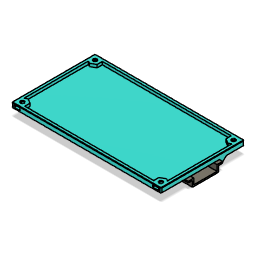
RelayBoardMount (Autodesk Fusion 360 design; units mm, degrees)
Autodesk Fusion 360 part; units mm, degrees
sketch "Skizze1" plane through (0, 0, 0) normal (1, 0, 0) x (0, 0, -1) in component "Rail"
  line L0 (-17.75, 0) -> (17.75, 0)
  line L1 (-13.5, -7.5) -> (13.5, -7.5)
  line L2 (0, -7.5) -> (0, 0) construction
  line L3 (-17.75, 0) -> (-17.75, -1.5)
  line L4 (17.75, 0) -> (17.75, -1.5)
  line L5 (13.5, -7.5) -> (13.5, -1.5)
  line L6 (13.5, -1.5) -> (17.75, -1.5)
  line L7 (-17.75, -1.5) -> (-13.5, -1.5)
  line L8 (-13.5, -1.5) -> (-13.5, -7.5)
  line L9 (-12, 0) -> (-12, -6)
  line L10 (-12, -6) -> (12, -6)
  line L11 (12, -6) -> (12, 0)
  dimension "d1" = 35.5
  dimension "d2" = 27
  dimension "d3" = 1.5
  dimension "d5" = 7.5
  dimension "d6" = 1.5
  dimension "d7" = 1.5
  dimension "d8" = 1.5
  constraint horizontal L0
  constraint midpoint L2.end L0
  constraint horizontal L1
  constraint midpoint L1 L2.start
  constraint coincident L2.end origin
  constraint vertical L2
  constraint perpendicular L0 L3
  constraint perpendicular L0 L4
  constraint perpendicular L1 L5
  constraint perpendicular L4 L6
  constraint perpendicular L5 L7
  constraint perpendicular L7 L8
  constraint equal L3 L4
  constraint coincident L0 L9.start
  constraint perpendicular L0 L9
  constraint perpendicular L5 L10
  constraint coincident L0 L11.end
  constraint perpendicular L0 L11
  measures "d1" distance of L0.start L0.end
  measures "d2" distance of L1.start L1.end
  measures "d3" distance of L0.end L4.end
  measures "d5" distance of L0 L1
  measures "d6" distance of L1 L10
  measures "d7" distance of L8 L9
  measures "d8" distance of L5 L11
extrude "Extrusion1" add sketch "Skizze1" along normal mid plane 160 contours L0 L1 L3 L4 L5 L6 L7 L8 L9 L10 L11 makes body 1 in component "Rail"
sketch "Skizze2" plane through (0, 0, 0) normal (0, 1, 0) x (1, 0, 0) in component "RelayBottom"
  line L0 (-74, 40) -> (74, 40)
  line L1 (74, 40) -> (74, -40)
  line L2 (74, -40) -> (-74, -40)
  line L3 (-74, -40) -> (-74, 40)
  line L4 (-74, 40) -> (74, -40) construction
  line L5 (74, 40) -> (-74, -40) construction
  line L6 (-77, 43) -> (77, 43)
  line L7 (77, 43) -> (77, -43)
  line L8 (77, -43) -> (-77, -43)
  line L9 (-77, -43) -> (-77, 43)
  circle A0 centre (-71.5, 37.5) radius 2
  line L10 (71.5, -37.5) -> (-71.5, -37.5) construction
  line L11 (-71.5, -37.5) -> (-71.5, 37.5) construction
  line L12 (-71.5, 37.5) -> (71.5, 37.5) construction
  line L13 (71.5, 37.5) -> (71.5, -37.5) construction
  line L14 (71.5, -37.5) -> (-71.5, 37.5) construction
  line L15 (-71.5, -37.5) -> (71.5, 37.5) construction
  circle A1 centre (71.5, 37.5) radius 2
  circle A2 centre (71.5, -37.5) radius 2
  circle A3 centre (-71.5, -37.5) radius 2
  line L16 (-68.5, 39.2321) -> (-71.5, 40.9641)
  line L17 (-71.5, 40.9641) -> (-74.5, 39.2321)
  line L18 (-74.5, 39.2321) -> (-74.5, 35.7679)
  line L19 (-74.5, 35.7679) -> (-71.5, 34.0359)
  line L20 (-71.5, 34.0359) -> (-68.5, 35.7679)
  line L21 (-68.5, 35.7679) -> (-68.5, 39.2321)
  line L22 (-68.5, 39.2321) -> (-68.5, 43)
  line L23 (-74.5, 39.2321) -> (-74.5, 43)
  line L24 (74.5, 35.7679) -> (74.5, 39.2321)
  line L25 (74.5, 39.2321) -> (71.5, 40.9641)
  line L26 (71.5, 40.9641) -> (68.5, 39.2321)
  line L27 (68.5, 39.2321) -> (68.5, 35.7679)
  line L28 (68.5, 35.7679) -> (71.5, 34.0359)
  line L29 (71.5, 34.0359) -> (74.5, 35.7679)
  line L30 (74.5, -35.7679) -> (71.5, -34.0359)
  line L31 (71.5, -34.0359) -> (68.5, -35.7679)
  line L32 (68.5, -35.7679) -> (68.5, -39.2321)
  line L33 (68.5, -39.2321) -> (71.5, -40.9641)
  line L34 (71.5, -40.9641) -> (74.5, -39.2321)
  line L35 (74.5, -39.2321) -> (74.5, -35.7679)
  line L36 (-68.5, -35.7679) -> (-71.5, -34.0359)
  line L37 (-71.5, -34.0359) -> (-74.5, -35.7679)
  line L38 (-74.5, -35.7679) -> (-74.5, -39.2321)
  line L39 (-74.5, -39.2321) -> (-71.5, -40.9641)
  line L40 (-71.5, -40.9641) -> (-68.5, -39.2321)
  line L41 (-68.5, -39.2321) -> (-68.5, -35.7679)
  line L42 (-74.5, -39.2321) -> (-74.5, -43)
  line L43 (-68.5, -39.2321) -> (-68.5, -43)
  line L44 (68.5, -39.2321) -> (68.5, -43)
  line L45 (74.5, -39.2321) -> (74.5, -43)
  line L46 (68.5, 39.2321) -> (68.5, 43)
  line L47 (74.5, 39.2321) -> (74.5, 43)
  line L48 (66.5, -39.2321) -> (66.5, -43)
  line L49 (66.5, -34.6132) -> (66.5, -39.2321)
  line L50 (71.5, -31.7265) -> (66.5, -34.6132)
  line L51 (76.5, -34.6132) -> (71.5, -31.7265)
  line L52 (76.5, -39.2321) -> (76.5, -34.6132)
  line L53 (76.5, -39.2321) -> (76.5, -43)
  line L54 (76.5, 39.2321) -> (76.5, 43)
  line L55 (76.5, 34.6132) -> (76.5, 39.2321)
  line L56 (71.5, 31.7265) -> (76.5, 34.6132)
  line L57 (66.5, 34.6132) -> (71.5, 31.7265)
  line L58 (66.5, 39.2321) -> (66.5, 34.6132)
  line L59 (66.5, 39.2321) -> (66.5, 43)
  line L60 (-66.5, 39.2321) -> (-66.5, 43)
  line L61 (-66.5, 34.6132) -> (-66.5, 39.2321)
  line L62 (-71.5, 31.7265) -> (-66.5, 34.6132)
  line L63 (-76.5, 34.6132) -> (-71.5, 31.7265)
  line L64 (-76.5, 39.2321) -> (-76.5, 34.6132)
  line L65 (-76.5, 39.2321) -> (-76.5, 43)
  line L66 (-76.5, -39.2321) -> (-76.5, -43)
  line L67 (-76.5, -34.6132) -> (-76.5, -39.2321)
  line L68 (-71.5, -31.7265) -> (-76.5, -34.6132)
  line L69 (-66.5, -34.6132) -> (-71.5, -31.7265)
  line L70 (-66.5, -39.2321) -> (-66.5, -34.6132)
  line L71 (-66.5, -39.2321) -> (-66.5, -43)
  point P0 (-71.5, 37.5)
  point P1 (71.5, 37.5)
  point P2 (71.5, -37.5)
  point P3 (-71.5, -37.5)
  dimension "d21" = 148
  dimension "d22" = 80
  dimension "d23" = -3
  dimension "d26" = 4
  dimension "d28" = 2.5
  dimension "d29" = 2.5
  dimension "d31" = 6
  dimension "d35" = 2
  dimension "d36" = 2
  dimension "d37" = -2
  dimension "d38" = 2
  constraint horizontal L0
  constraint perpendicular L0 L1
  constraint parallel L0 L2
  constraint parallel L1 L3
  constraint coincident L4 origin
  constraint coincident L5 origin
  constraint horizontal L10
  constraint perpendicular L10 L11
  constraint parallel L10 L12
  constraint parallel L11 L13
  constraint coincident L14 origin
  constraint coincident L15 origin
  constraint coincident P0 A0.centre
  constraint coincident P1 L12.end
  constraint coincident P2 L10.start
  constraint coincident P3 L10.end
  constraint equal A0 A3
  constraint equal A0 A2
  constraint equal A0 A1
  constraint coincident L6 L22.end
  constraint perpendicular L6 L22
  constraint coincident L6 L23.end
  constraint perpendicular L6 L23
  constraint collinear L21 L22
  constraint equal L21 L26
  constraint equal L21 L32
  constraint equal L21 L41
  constraint coincident L8 L42.end
  constraint parallel L38 L42
  constraint perpendicular L8 L42
  constraint coincident L8 L43.end
  constraint perpendicular L8 L43
  constraint coincident L8 L44.end
  constraint perpendicular L8 L44
  constraint collinear L32 L44
  constraint coincident L8 L45.end
  constraint perpendicular L8 L45
  constraint coincident L6 L46.end
  constraint perpendicular L6 L46
  constraint collinear L27 L46
  constraint coincident L6 L47.end
  constraint perpendicular L6 L47
  measures "d21" distance of L1.end L2.end
  measures "d22" distance of L0.end L1.end
  measures "d26" diameter of A0
  measures "d28" distance of L1 L13
  measures "d29" distance of L2 L10
  measures "d31" distance of L18 L21
extrude "Extrusion2" add sketch "Skizze2" along normal blind 2 separate body contours L0 L3 L6 L16 L17 L22 L23 | L0 L3 L17 | L0 L16 L17 | L0 L3 L16 L17 L19 L20 L21 | L3 L17 L18 L19 | L0 L16 L22 | L0 L3 L19 L20 L21 L22 L60 L61 L62 L63 | L3 L6 L18 L19 L23 L63 L64 L65 | L0 L6 L22 L60 | L0 L1 L2 L3 L48 L49 L50 L51 L56 L57 L58 L59 L60 L61 L62 L63 L68 L69 L70 L71 | L3 L6 L8 L9 L63 L64 L65 L66 L67 L68 | L0 L6 L59 L60 | L2 L3 L36 L37 L41 L43 L68 L69 L70 L71 | L3 L8 L37 L38 L42 L66 L67 L68 | L0 L6 L46 L59 | L0 L1 L27 L28 L29 L46 L56 L57 L58 L59 | L2 L3 L36 L37 L39 L40 L41 | L3 L37 L38 L39 | L0 L1 L6 L25 L26 L46 L47 | L0 L26 L46 | L2 L3 L39 | L2 L3 L8 L39 L40 L42 L43 | L0 L25 L26 | L0 L1 L25 L26 L27 L28 L29 | L2 L39 L40 | L0 L1 L25 | L1 L6 L24 L29 L47 L54 L55 L56 | L2 L40 L43 | L2 L8 L43 L71 | L2 L8 L48 L71 | L1 L24 L25 L29 | L1 L6 L7 L8 L51 L52 L53 L54 L55 L56 | L1 L2 L30 L31 L32 L44 L48 L49 L50 L51 | L2 L8 L44 L48 | L1 L8 L30 L35 L45 L51 L52 L53 | L2 L33 L44 | L1 L2 L8 L33 L34 L44 L45 | L1 L30 L34 L35 | L1 L2 L30 L31 L32 L33 L34 | L2 L33 L34 | L1 L2 L34 | A0 | A1 | A2 | A3 makes body 2 in component "RelayBottom"
extrude "Extrusion4" add sketch "Skizze2" along normal blind 3 from surface at 2 contours L0 L3 L6 L16 L17 L22 L23 | L0 L3 L17 | L0 L16 L17 | L0 L3 L16 L17 L19 L20 L21 | L3 L17 L18 L19 | L0 L16 L22 | L0 L3 L19 L20 L21 L22 L60 L61 L62 L63 | L3 L6 L18 L19 L23 L63 L64 L65 | L0 L6 L22 L60 | L3 L6 L8 L9 L63 L64 L65 L66 L67 L68 | L0 L6 L59 L60 | L2 L3 L36 L37 L41 L43 L68 L69 L70 L71 | L3 L8 L37 L38 L42 L66 L67 L68 | L0 L6 L46 L59 | L0 L1 L27 L28 L29 L46 L56 L57 L58 L59 | L2 L3 L36 L37 L39 L40 L41 | L3 L37 L38 L39 | L0 L1 L6 L25 L26 L46 L47 | L0 L26 L46 | L2 L3 L39 | L2 L3 L8 L39 L40 L42 L43 | L0 L25 L26 | L0 L1 L25 L26 L27 L28 L29 | L2 L39 L40 | L0 L1 L25 | L1 L6 L24 L29 L47 L54 L55 L56 | L2 L40 L43 | L2 L8 L43 L71 | L2 L8 L48 L71 | L1 L24 L25 L29 | L1 L6 L7 L8 L51 L52 L53 L54 L55 L56 | L1 L2 L30 L31 L32 L44 L48 L49 L50 L51 | L2 L8 L44 L48 | L1 L8 L30 L35 L45 L51 L52 L53 | L2 L33 L44 | L1 L2 L8 L33 L34 L44 L45 | L1 L30 L34 L35 | L1 L2 L30 L31 L32 L33 L34 | L2 L33 L34 | L1 L2 L34 bodies 2 in component "RelayBottom"
extrude "Extrusion3" cut sketch "Skizze2" along normal blind 2.5 from surface at 1.5 contours L0 L3 L6 L16 L17 L22 L23 | L0 L3 L17 | L0 L16 L17 | L0 L3 L16 L17 L19 L20 L21 | L3 L17 L18 L19 | L0 L16 L22 | L2 L3 L36 L37 L39 L40 L41 | L3 L37 L38 L39 | L0 L1 L6 L25 L26 L46 L47 | L0 L26 L46 | L2 L3 L39 | L2 L3 L8 L39 L40 L42 L43 | L0 L25 L26 | L0 L1 L25 L26 L27 L28 L29 | L2 L39 L40 | L0 L1 L25 | L2 L40 L43 | L1 L24 L25 L29 | L2 L33 L44 | L1 L2 L8 L33 L34 L44 L45 | L1 L30 L34 L35 | L1 L2 L30 L31 L32 L33 L34 | L2 L33 L34 | L1 L2 L34 | A0 | A1 | A2 | A3 bodies 2 in component "RelayBottom"
fillet "Abrundung2" radius 1 4 edges at (-77, 2.5, 43) (77, 2.5, 43) (77, 2.5, -43) (-77, 2.5, -43) on bodies 2 in component "RelayBottom"
sketch "Skizze3" plane through (0, 0, 0) normal (1, 0, 0) x (0, 0, -1) in component "RelayBottom"
  line L0 (-17.75, -1.5) -> (-17.75, 0)
  line L1 (-17.75, 0) -> (-12, 0)
  line L2 (-12, 0) -> (-12, -6)
  line L3 (-12, -6) -> (12, -6)
  line L4 (12, -6) -> (12, 0)
  line L5 (12, 0) -> (17.75, 0)
  line L6 (17.75, 0) -> (17.75, -1.5)
  line L7 (17.75, -1.5) -> (13.5, -1.5)
  line L8 (13.5, -1.5) -> (13.5, -7.5)
  line L9 (13.5, -7.5) -> (-13.5, -7.5)
  line L10 (-13.5, -7.5) -> (-13.5, -1.5)
  line L11 (-13.5, -1.5) -> (-17.75, -1.5)
  line L12 (14.5, -5) -> (19.75, -5)
  line L13 (19.75, -5) -> (24.75, 0)
  line L14 (14.5, -5) -> (14.5, -2)
  line L15 (14.5, -2) -> (17.75, -2)
  line L16 (17.75, -2) -> (17.75, -1.5)
  line L17 (-42, 0) -> (42, 0)
  line L18 (-42, 0) -> (-43, 0)
  line L19 (43, 0) -> (42, 0)
  line L20 (-18.25, 0) -> (-18.25, -1.7)
  line L21 (-18.25, -1.7) -> (-16.95, -1.7)
  line L22 (-16.95, -1.7) -> (-16.95, -3.7)
  line L23 (-16.95, -3.7) -> (-20.25, -3.7)
  line L24 (-20.25, -3.7) -> (-23.95, 0)
  point P0 (-43, 0)
  dimension "d45" = 3
  dimension "d46" = 1
  dimension "d47" = 0.5
  dimension "d64" = 45
  dimension "d65" = 2
  dimension "d67" = 45
  dimension "d68" = 2
  dimension "d69" = 2
  dimension "d70" = 0.5
  dimension "d71" = 0.8
  dimension "d78" = 0.2
  constraint perpendicular L12 L14
  constraint perpendicular L14 L15
  constraint coincident L6.end L7.start
  constraint perpendicular L15 L16
  constraint coincident L13.end L17
  constraint coincident L17 L20.start
  constraint perpendicular L17 L20
  constraint perpendicular L20 L21
  constraint perpendicular L21 L22
  constraint perpendicular L22 L23
  constraint coincident L17 L24.end
  measures "d45" distance of L12.start L14.end
  measures "d46" distance of L8 L14
  measures "d47" distance of L7 L15
  measures "d64" angle of L17 L24
  measures "d65" distance of L6 L12.end
  measures "d67" angle of L13 L17
  measures "d68" distance of L21 L23
  measures "d69" distance of L20 L23.end
  measures "d70" distance of L0 L20
  measures "d71" distance of L0 L22
  measures "d78" distance of L11 L21
ref_plane "Arbeitsebene1" through (-67, 2.5, 0) normal (-1, 0, 0) x (0, 0, 1) in component "RelayBottom"
ref_plane "Arbeitsebene2" through (67, 2.5, 0) normal (1, 0, 0) x (0, 0, -1) in component "RelayBottom"
extrude "Extrusion5" add sketch "Skizze3" along normal up to surface (77 mm away) and the other way up to surface (77 mm away) contours L6 L12 L13 L14 L15 L16 L17 bodies 2 in component "RelayBottom"
extrude "Extrusion6" add sketch "Skizze3" against normal blind 10 from surface at 67 contours L17 L20 L21 L22 L23 L24 bodies 2 in component "RelayBottom"
extrude "Extrusion7" add sketch "Skizze3" along normal blind 10 from surface at -67 contours L17 L20 L21 L22 L23 L24 bodies 2 in component "RelayBottom"
chamfer "Fase2" distance 0.5 angle 45 1 edges at (0, -2, -14.5) on bodies 2 in component "RelayBottom"
fillet "Abrundung3" radius 0.75 4 edges at (62, -1.7, 16.95) (62, -3.7, 16.95) (-62, -3.7, 16.95) (-62, -1.7, 16.95) on bodies 2 in component "RelayBottom"
fillet "Abrundung3" radius 2 3 edges at (-62, -3.7, 20.25) (62, -3.7, 20.25) (0, -5, -19.75) on bodies 2 in component "RelayBottom"
fillet "Abrundung3" radius 2 3 edges at (-62, 0, 23.95) (62, 0, 23.95) (0, 0, -24.75) on bodies 2 in component "RelayBottom"
chamfer "Fase1" distance 0.4 angle 45 8 edges at (-77, 5, 0) (-76.7071, 5, 42.7071) (0, 5, 43) (76.7071, 5, 42.7071) (77, 5, 0) (76.7071, 5, -42.7071) (0, 5, -43) (-76.7071, 5, -42.7071) on bodies 2 in component "RelayBottom"
chamfer "Fase1" distance 0.4 angle 45 18 edges at (-77, 0, 12.125) (77, 0, 12.125) (76.7071, 0, 42.7071) (0, 0, 43) (-76.7071, 0, 42.7071) (-77, 0, -33.7892) (-76.7071, 0, -42.7071) (0, 0, -43) (76.7071, 0, -42.7071) (77, 0, -33.7892) (77, -0.1522, -24.8131) (77, -2.5, -22.25) (77, -4.8478, -19.6869) (77, -5, -16.7108) (-77, -5, -16.7108) (-77, -4.8478, -19.6869) (-77, -2.5, -22.25) (-77, -0.1522, -24.8131) on bodies 2 in component "RelayBottom"
component "Rail" placed x (1, 0, 0) y (0, 1, 0) z (0, 0, 1) at (0, 0, 0)
component "RelayBottom" placed x (1, 0, 0) y (0, 1, 0) z (0, 0, 1) at (0, 0, 0)
